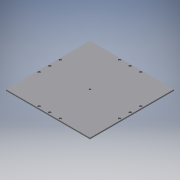
# Autodesk Inventor part: 00_LED-ARRAY
Saved by Autodesk Inventor 2019 (Build 230136000, 136)
## iProperties
Created: 2017-05-04
Part Number: 00_LED-ARRAY
Material: Generisch
Document SubType Name: Modeling
Designer: diederichbenedict
Density: 1 g/cm^3
Appearance: Vorgabe
Mass: 4.18553 g
Surface Area: 87.1118 cm^2
Volume: 4.18553 cm^3
Author: diederichbenedict
Autodesk Inventor part; units mm, degrees
ref_plane "YZ Plane" through (0, 0, 0) normal (1, 0, 0) x (0, 1, 0)
ref_plane "XZ Plane" through (0, 0, 0) normal (0, 1, 0) x (-1, 0, 0)
ref_plane "XY Plane" through (0, 0, 0) normal (0, 0, 1) x (1, 0, 0)
ref_plane "Arbeitsebene1" through (0, 0, 50) normal (0, 0, 1) x (1, 0, 0)
sketch "Skizze1" plane through (0, 0, 50) normal (0, 0, 1) x (1, 0, 0)
  circle A0 centre (0, -2) radius 0.75 projected
  line L0 (32.5, 30.5) -> (-32.5, 30.5)
  line L1 (-32.5, 30.5) -> (-32.5, -34.5)
  line L2 (-32.5, -34.5) -> (32.5, -34.5)
  line L3 (32.5, -34.5) -> (32.5, 30.5)
  line L4 (32.5, 30.5) -> (-32.5, -34.5) construction
  line L5 (-32.5, 30.5) -> (32.5, -34.5) construction
  point P0 (0, 0)
  dimension "d0" = 65
  dimension "d1" = 65
  constraints: 12 end point, 2 midpoint, 2 parallel, 1 horizontal, 1 perpendicular
  measures "d0" distance of L2.end L1.end
  measures "d1" distance of L1.end L0.end
extrude "Extrusion1" add sketch "Skizze1" along normal blind 1
sketch "Skizze2" plane through (0, 0, 50) normal (0, 0, 1) x (1, 0, 0)
  circle A0 centre (0, -2) radius 0.75 projected
  line L0 (32.5, 30.5) -> (-32.5, 30.5) projected
  line L1 (-32.5, 30.5) -> (-32.5, -34.5) projected
  line L2 (-32.5, -34.5) -> (32.5, -34.5) projected
  line L3 (32.5, -34.5) -> (32.5, 30.5) projected
  circle A1 centre (0, -33.1) radius 1
  circle A2 centre (0, 29.1) radius 1
  circle A3 centre (8.2, -33.1) radius 1
  circle A4 centre (-8.2, -33.1) radius 1
  circle A5 centre (-8.2, 29.1) radius 1
  circle A6 centre (8.2, 29.1) radius 1
  point P0 (0, 0)
  point P1 (3.8, 10.2517)
  dimension "d4" = 2
  dimension "d5" = 2
  dimension "d6" = 1.4
  dimension "d7" = 1.4
  dimension "d8" = 2
  dimension "d9" = 2
  dimension "d10" = 2
  dimension "d11" = 2
  constraints: 6 centre point, 1 other
  measures "d4" diameter of A1
  measures "d5" diameter of A2
  measures "d6" distance from line of L0 A2.centre
  measures "d7" distance from line of A1.centre L2
  measures "d8" diameter of A3
  measures "d9" diameter of A4
  measures "d10" diameter of A5
  measures "d11" diameter of A6
extrude "Extrusion2" cut sketch "Skizze2" along normal blind 1 contours A1 | A2 | A3 | A4 | A5 | A6
pattern_circular "Runde Anordnung1" count 4 over 360 about axis through (0, -2, 50) along (0, 0, 1) of "Extrusion2"
